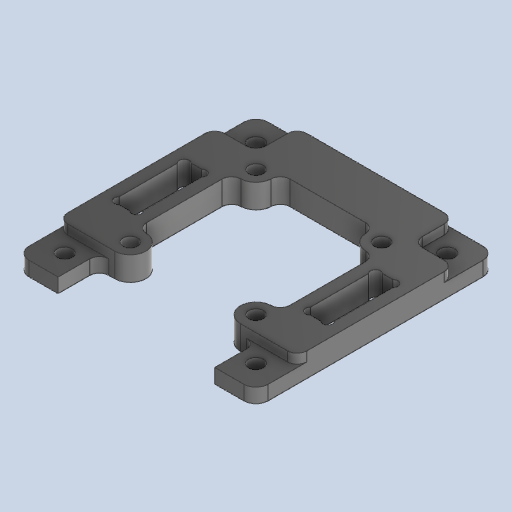
# Autodesk Inventor part: Camera_root_frame_e-CAM50_CUNX
Saved by Autodesk Inventor 2022 (Build 260153000, 153)
## iProperties
Part Number: Camera_root_frame_e-CAM50_CUNX
Material: アセタール樹脂、黒
Document SubType Name: Modeling
Designer: Masato Kubotera
Density: 1.425 g/cm^3
Appearance: 滑らか - 黒
Description: POM T5
Mass: 7.52062 g
Surface Area: 43.8895 cm^2
Volume: 5.27763 cm^3
Author: Masato Kubotera
Autodesk Inventor part; units mm, degrees
ref_plane "YZ Plane" through (0, 0, 0) normal (1, 0, 0) x (0, 1, 0)
ref_plane "XZ Plane" through (0, 0, 0) normal (0, 1, 0) x (-1, 0, 0)
ref_plane "XY Plane" through (0, 0, 0) normal (0, 0, 1) x (1, 0, 0)
derived "e-CAM50_CUNX.ipt"
sketch "スケッチ1" plane through (0, 0, 0) normal (0, 0, 1) x (1, 0, 0)
  line L0 (15, 15) -> (-15, 15) construction
  line L1 (-15, 15) -> (-15, -15) construction
  line L2 (-15, -15) -> (15, -15) construction
  line L3 (15, -15) -> (15, 15) construction
  line L4 (15, 15) -> (-15, -15) construction
  line L5 (-15, 15) -> (15, -15) construction
  line L6 (-13.14, 13.14) -> (13.14, 13.14) construction
  line L7 (13.14, 13.14) -> (13.14, -13.14) construction
  line L8 (13.14, -13.14) -> (-13.14, -13.14) construction
  line L9 (-13.14, -13.14) -> (-13.14, 13.14) construction
  line L10 (-13.14, 13.14) -> (13.14, -13.14) construction
  line L11 (13.14, 13.14) -> (-13.14, -13.14) construction
  circle A0 centre (-13.14, -13.14) radius 1.1 construction
  line L12 (-15, 0) -> (15, 0) construction
  line L13 (0, 15) -> (0, -15) construction
  circle A1 centre (-13.14, 13.14) radius 1.1 construction
  circle A2 centre (13.14, 13.14) radius 1.1 construction
  circle A3 centre (13.14, -13.14) radius 1.1 construction
  circle A4 centre (-13.14, -13.14) radius 2 construction
  circle A5 centre (-13.14, 13.14) radius 2 construction
  circle A6 centre (13.14, -13.14) radius 2 construction
  circle A7 centre (13.14, 13.14) radius 2 construction
  circle A8 centre (0, 0) radius 8.5 construction
  line L14 (-7, 8) -> (7, 8)
  line L15 (8, 7) -> (8, -7)
  line L16 (7, -8) -> (-7, -8)
  line L17 (-8, -7) -> (-8, 7)
  line L18 (-8, 8) -> (8, -8) construction
  line L19 (8, 8) -> (-8, -8) construction
  arc A9 (-7, 8) -> (-8, 7) centre (-7, 7) ccw
  arc A10 (-8, -7) -> (-7, -8) centre (-7, -7) ccw
  arc A11 (7, -8) -> (8, -7) centre (7, -7) ccw
  arc A12 (8, 7) -> (7, 8) centre (7, 7) ccw
  arc A13 (-10, 2) -> (-10, -2) centre (-10, 0) ccw
  line L20 (-10, 2) -> (-8, 2)
  line L21 (-10, -2) -> (-8, -2)
  line L22 (10, 2) -> (8, 2)
  arc A14 (10, -2) -> (10, 2) centre (10, 0) ccw
  line L23 (10, -2) -> (8, -2)
  line L24 (-8.2717, 14) -> (8.2717, 14)
  line L25 (14, 8.2717) -> (14, -8.2717)
  line L26 (8.2717, -14) -> (-8.2717, -14)
  line L27 (-14, -8.2717) -> (-14, 8.2717)
  line L28 (-14, 14) -> (14, -14) construction
  line L29 (14, 14) -> (-14, -14) construction
  arc A15 (12.456, -10.219) -> (10.219, -12.456) centre (13.14, -13.14) ccw
  arc A16 (-10.219, -12.456) -> (-12.456, -10.219) centre (-13.14, -13.14) ccw
  arc A17 (-12.456, 10.219) -> (-10.219, 12.456) centre (-13.14, 13.14) ccw
  arc A18 (10.219, 12.456) -> (12.456, 10.219) centre (13.14, 13.14) ccw
  arc A19 (8.2717, -14) -> (10.219, -12.456) centre (8.2717, -12) ccw
  arc A20 (12.456, -10.219) -> (14, -8.2717) centre (12, -8.2717) ccw
  arc A21 (14, 8.2717) -> (12.456, 10.219) centre (12, 8.2717) ccw
  arc A22 (10.219, 12.456) -> (8.2717, 14) centre (8.2717, 12) ccw
  arc A23 (-8.2717, 14) -> (-10.219, 12.456) centre (-8.2717, 12) ccw
  arc A24 (-12.456, 10.219) -> (-14, 8.2717) centre (-12, 8.2717) ccw
  arc A25 (-14, -8.2717) -> (-12.456, -10.219) centre (-12, -8.2717) ccw
  arc A26 (-10.219, -12.456) -> (-8.2717, -14) centre (-8.2717, -12) ccw
  point P0 (8, 2)
  point P1 (8, -2)
  point P2 (14, -10.2659)
  point P3 (10.2659, -14)
  point P4 (-14, -10.2659)
  point P5 (-10.2659, -14)
  point P6 (-10.2659, 14)
  point P7 (-14, 10.2659)
  point P8 (14, 10.2659)
  point P9 (10.2659, 14)
sketch "スケッチ2" plane through (0, 0, 0) normal (0, 0, 1) x (1, 0, 0)
  line L0 (-22.5, 25) -> (22.5, 25)
  line L1 (25, 22.5) -> (25, -22.5)
  line L2 (22.5, -25) -> (-22.5, -25)
  line L3 (-25, -22.5) -> (-25, 22.5)
  line L4 (-25, 25) -> (25, -25) construction
  line L5 (25, 25) -> (-25, -25) construction
  arc A0 (-22.5, 25) -> (-25, 22.5) centre (-22.5, 22.5) ccw
  arc A1 (-25, -22.5) -> (-22.5, -25) centre (-22.5, -22.5) ccw
  arc A2 (22.5, -25) -> (25, -22.5) centre (22.5, -22.5) ccw
  arc A3 (25, 22.5) -> (22.5, 25) centre (22.5, 22.5) ccw
  line L6 (-25, -22.5) -> (25, -22.5) construction
  line L7 (25, -22.5) -> (25, -17.5)
  line L8 (25, -17.5) -> (-25, -17.5) construction
  line L9 (-25, -17.5) -> (-25, -22.5) construction
  line L10 (-25, -22.5) -> (25, -17.5) construction
  line L11 (25, -22.5) -> (-25, -17.5) construction
  line L12 (-25, -20) -> (25, -20) construction
  line L13 (0, 15) -> (0, -15) construction
  circle A4 centre (-20, -20) radius 1.6
  circle A5 centre (20, -20) radius 1.6
  line L14 (-15, 0) -> (15, 0) construction
  circle A6 centre (-20, 20) radius 1.6
  circle A7 centre (20, 20) radius 1.6
  circle A8 centre (13.14, 13.14) radius 1.1 projected
  circle A9 centre (13.14, -13.14) radius 1.1 projected
  circle A10 centre (-13.14, -13.14) radius 1.1 projected
  circle A11 centre (-13.14, 13.14) radius 1.1 projected
  circle A12 centre (-13.14, -13.14) radius 1.55
  circle A13 centre (13.14, -13.14) radius 1.55
  circle A14 centre (13.14, 13.14) radius 1.55
  circle A15 centre (-13.14, 13.14) radius 1.55
  line L15 (-15, -15) -> (15, -15) construction
  line L16 (-15, 15) -> (-15, -15) construction
  line L17 (-15, -7.8919) -> (-15, 0)
  line L18 (0, -15) -> (-7.8919, -15)
  arc A16 (-9.8912, -13.0533) -> (-13.0533, -9.8912) centre (-13.14, -13.14) ccw
  arc A17 (-9.8912, -13.0533) -> (-7.8919, -15) centre (-7.8919, -13) ccw
  arc A18 (-15, -7.8919) -> (-13.0533, -9.8912) centre (-13, -7.8919) ccw
  line L19 (-15, 7.8919) -> (-15, 0)
  line L20 (0, 15) -> (-7.8919, 15)
  arc A19 (-13.0533, 9.8912) -> (-9.8912, 13.0533) centre (-13.14, 13.14) ccw
  arc A20 (-7.8919, 15) -> (-9.8912, 13.0533) centre (-7.8919, 13) ccw
  arc A21 (-13.0533, 9.8912) -> (-15, 7.8919) centre (-13, 7.8919) ccw
  line L21 (0, -15) -> (7.8919, -15)
  arc A22 (16.39, -13.14) -> (9.8912, -13.0533) centre (13.14, -13.14) ccw
  arc A23 (7.8919, -15) -> (9.8912, -13.0533) centre (7.8919, -13) ccw
  arc A24 (9.8912, 13.0533) -> (7.8919, 15) centre (7.8919, 13) ccw
  line L22 (0, 15) -> (7.8919, 15)
  line L23 (-7.5, -22.5) -> (7.5, -22.5) construction
  line L24 (7.5, -22.5) -> (7.5, -17.5) construction
  line L25 (7.5, -17.5) -> (-7.5, -17.5) construction
  line L26 (-7.5, -17.5) -> (-7.5, -22.5) construction
  line L27 (-7.5, -22.5) -> (7.5, -17.5) construction
  line L28 (7.5, -22.5) -> (-7.5, -17.5) construction
  line L29 (-6.0651, -22.55) -> (6.0651, -22.55)
  line L30 (6.0651, -17.45) -> (-6.0651, -17.45)
  arc A25 (-7.55, -21.0651) -> (-6.0651, -22.55) centre (-6.8075, -21.8075) ccw
  arc A26 (-6.0651, -17.45) -> (-7.55, -18.9349) centre (-6.8075, -18.1925) ccw
  arc A27 (6.0651, -22.55) -> (7.55, -21.0651) centre (6.8075, -21.8075) ccw
  arc A28 (7.55, -18.9349) -> (6.0651, -17.45) centre (6.8075, -18.1925) ccw
  line L31 (-7.55, -22.5) -> (-7.55, -22.55)
  line L32 (-7.55, -18.9349) -> (-7.55, -21.0651)
  line L33 (7.55, -21.0651) -> (7.55, -18.9349)
  line L34 (-6.0651, 22.55) -> (6.0651, 22.55)
  line L35 (6.0651, 17.45) -> (-6.0651, 17.45)
  arc A29 (-6.0651, 22.55) -> (-7.55, 21.0651) centre (-6.8075, 21.8075) ccw
  arc A30 (-7.55, 18.9349) -> (-6.0651, 17.45) centre (-6.8075, 18.1925) ccw
  arc A31 (6.0651, 17.45) -> (7.55, 18.9349) centre (6.8075, 18.1925) ccw
  arc A32 (7.55, 21.0651) -> (6.0651, 22.55) centre (6.8075, 21.8075) ccw
  line L36 (-7.55, 18.9349) -> (-7.55, 21.0651)
  line L37 (7.55, 21.0651) -> (7.55, 18.9349)
  arc A33 (-16.39, -18.39) -> (-18.39, -16.39) centre (-18.39, -18.39) ccw
  line L38 (-16.39, -18.39) -> (-16.39, -23)
  arc A34 (-16.3897, -22.9663) -> (-14.39, -25) centre (-14.39, -23) ccw
  line L39 (-16.39, 18.39) -> (-16.39, 23)
  arc A35 (-14.39, 25) -> (-16.3897, 22.9663) centre (-14.39, 23) ccw
  line L40 (16.39, -13.14) -> (16.39, -23)
  arc A36 (14.39, -25) -> (16.3897, -22.9663) centre (14.39, -23) ccw
  arc A37 (16.3897, 22.9663) -> (14.39, 25) centre (14.39, 23) ccw
  line L41 (15, 0) -> (-15, 0) construction
  arc A38 (-25, -14.39) -> (-23, -16.39) centre (-23, -14.39) ccw
  line L42 (-23, -16.39) -> (-18.39, -16.39)
  arc A39 (-18.39, 16.39) -> (-16.39, 18.39) centre (-18.39, 18.39) ccw
  arc A40 (-23, 16.39) -> (-25, 14.39) centre (-23, 14.39) ccw
  line L43 (-23, 16.39) -> (-18.39, 16.39)
  arc A41 (16.39, -14.39) -> (18.39, -16.39) centre (18.39, -14.39) ccw
  arc A42 (9.8912, 13.0533) -> (16.39, 13.14) centre (13.14, 13.14) ccw
  line L44 (16.39, 13.14) -> (16.39, 23)
  arc A43 (18.39, 16.39) -> (16.39, 14.39) centre (18.39, 14.39) ccw
  line L45 (18.39, -16.39) -> (25, -16.39)
  line L46 (18.39, 16.39) -> (25, 16.39)
  point P0 (0, 0)
  point P1 (0, -20)
  point P2 (0, -20)
  point P3 (-10.4749, -15)
  point P4 (-15, 7.8919)
  point P5 (7.8919, -15)
  point P6 (-7.8919, -15)
  point P7 (-16.9758, -16.9758)
  point P8 (14.39, -25)
  point P9 (14.39, 25)
  point P10 (-14.39, 25)
  point P11 (-25, 14.39)
  point P12 (-7.5968, -22.5)
  point P13 (7.5968, -22.5)
  point P14 (7.5968, 22.5)
  point P15 (-7.5968, 22.5)
  dimension "d1" = 50
  dimension "d2" = 50
  dimension "d3" = 2.5
  dimension "d7" = 5
  dimension "d8" = 5
  dimension "d9" = 3.2
  dimension "d10" = 5
  dimension "d12" = 3.1
  dimension "d20" = 2
  dimension "d21" = 40
  dimension "d23" = 12.5
  dimension "d24" = 15
  dimension "d27" = 0.05
  dimension "d28" = 1.05
  dimension "d30" = 0.05
  dimension "d39" = 2
  dimension "d40" = 2
  dimension "d41" = 3.61
  dimension "d46" = 15
  dimension "d59" = 3.61
  dimension "d60" = 2
  dimension "d61" = 3.25
  dimension "d71" = 26.28
  dimension "d72" = 32.78
  constraints: 86 end point, 71 point on circle, 64 symmetric about line, 40 centre point, 25 point on line, 20 tangent, 10 parallel, 9 midpoint, 6 perpendicular, 5 coincident, 4 equal radius, 4 horizontal, 2 collinear, 1 vertical, 26 other
  measures "d1" distance of L4.end L5.end
  measures "d2" distance of L5.start L4.end
  measures "d3" radius of A0
  measures "d7" distance of L7.end L6.end
  measures "d8" distance from line of L5.end L12
  measures "d9" diameter of A4
  measures "d10" distance of L12.start A4.centre
  measures "d12" diameter of A12
  measures "d20" radius of A17
  measures "d21" distance of A6.centre A4.centre
  measures "d23" horizontal distance of L23.start A4.centre
  measures "d24" distance of L23.end L23.start
  measures "d27" distance between parallel lines of L29 L23
  measures "d28" radius of A25
  measures "d30" distance between parallel lines of L26 L32
  measures "d39" radius of A34
  measures "d40" radius of A33
  measures "d41" horizontal distance of L38.end A4.centre
  measures "d46" distance of point (0, 0) L14.start
  measures "d59" distance from line of A4.centre L42
  measures "d60" radius of A38
  measures "d61" radius of A16
  measures "d71" distance of A9.centre A10.centre
  measures "d72" distance between parallel lines of L40 L38
extrude "押し出し1" add sketch "スケッチ2" along normal blind 5 contours L0 A37 L44 A42 A24 L22 L20 A20 A19 A21 L19 L17 A18 A16 A17 L18 L21 A23 A22 L40 A36 L2 A34 L38 A33 L42 A38 L3 A40 L43 A39 L39 A35
extrude "押し出し2" add sketch "スケッチ2" along normal blind 3 contours L0 A35 L39 A39 L43 A40 L3 A0 | L0 A3 L1 L46 A43 L44 A37 | A38 L42 A33 L38 A34 L2 A1 L3 | L1 A2 L2 A36 L40 A41 L45
equation "\"d27\" = d26"
equation "\"d40\" = d39"
equation "\"d26\" = 0.05"
